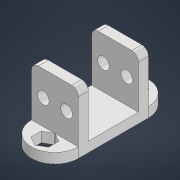
# Autodesk Inventor part: Stationary Bracket
Saved by Autodesk Inventor 2022 (Build 260153000, 153)
## iProperties
Created: 2022-01-30
Part Number: Stationary Bracket
Material: Generic
Document SubType Name: Modeling
Designer: izack
Density: 1 g/cm^3
Appearance: Default
Author: izack
## iProperties of the stored document Stationary Bracket_3DPrint.ipt
Part Number: Stationary Bracket_3DPrint
Material: Generic
Document SubType Name: Modeling
Designer: izack
Appearance: Default
Author: izack
Autodesk Inventor part; units mm, degrees
ref_plane "YZ Plane" through (0, 0, 0) normal (1, 0, 0) x (0, 1, 0)
ref_plane "XZ Plane" through (0, 0, 0) normal (0, 1, 0) x (-1, 0, 0)
ref_plane "XY Plane" through (0, 0, 0) normal (0, 0, 1) x (1, 0, 0)
sketch "Sketch1" plane through (0, 0, 0) normal (0, 1, 0) x (-1, 0, 0)
  line L0 (-7, 10.5) -> (7, 10.5)
  line L1 (7, 10.5) -> (7, -10.5)
  line L2 (7, -10.5) -> (-7, -10.5)
  line L3 (-7, -10.5) -> (-7, 10.5)
  line L4 (-7, 10.5) -> (7, -10.5) construction
  line L5 (7, 10.5) -> (-7, -10.5) construction
  line L6 (-7, 7.5) -> (7, 7.5)
  line L7 (7, 7.5) -> (7, -7.5)
  line L8 (7, -7.5) -> (-7, -7.5)
  line L9 (-7, -7.5) -> (-7, 7.5)
  line L10 (-7, 7.5) -> (7, -7.5) construction
  line L11 (7, 7.5) -> (-7, -7.5) construction
  line L12 (7, 0) -> (-7, 0) construction
  circle A0 centre (3.5, 0) radius 1.25
  circle A1 centre (-3.5, 0) radius 1.25
  point P0 (0, 0)
  dimension "d0" = 14
  dimension "d1" = 21
  dimension "d2" = 15
  dimension "d3" = 2.5
  dimension "d4" = 2.5
  dimension "d5" = 3.5
  dimension "d6" = 3.5
  constraints: 26 end point, 6 midpoint, 4 parallel, 3 point on line, 2 centre point, 2 horizontal, 2 perpendicular
  measures "d0" distance of L1.end L2.end
  measures "d1" distance of L0.end L1.end
  measures "d2" distance of L6.end L7.end
  measures "d3" diameter of A0
  measures "d4" diameter of A1
  measures "d5" distance from line of L1 A0.centre
  measures "d6" distance from line of L3 A1.centre
extrude "Extrusion1" add sketch "Sketch1" along normal blind 3
sketch "Sketch2" plane through (0, 0, 0) normal (0, -1, 0) x (1, 0, 0)
  line L0 (7, -10.5) -> (-7, -10.5) projected
  line L1 (7, 10.5) -> (7, -10.5) projected
  line L2 (-7, -10.5) -> (7, -10.5)
  line L3 (7, -10.5) -> (7, -7.5)
  line L4 (7, -7.5) -> (-7, -7.5)
  line L5 (-7, -7.5) -> (-7, -10.5)
  line L6 (-7, 10.5) -> (7, 10.5) projected
  line L7 (-7, 10.5) -> (7, 10.5)
  line L8 (7, 10.5) -> (7, 7.5)
  line L9 (7, 7.5) -> (-7, 7.5)
  line L10 (-7, 7.5) -> (-7, 10.5)
  point P0 (0, 0)
  dimension "d9" = 3
  dimension "d10" = 3
  constraints: 16 end point, 4 parallel, 2 horizontal, 2 perpendicular, 2 point on line
  measures "d9" distance of L3.end L2.end
  measures "d10" distance of L7.end L8.end
extrude "Extrusion2" add sketch "Sketch2" along normal blind 18
sketch "Sketch3" plane through (-7, 3, 10.5) normal (0, 0, 1) x (1, 0, 0)
  line L0 (14, -3) -> (0, -3) projected
  line L1 (0, -3) -> (14, -3)
  line L2 (0, -3) -> (0, -21) construction
  line L3 (0, -10.5) -> (14, -10.5) construction
  circle A0 centre (3.5, -10.5) radius 1.75
  circle A1 centre (10.5, -10.5) radius 1.75
  line L4 (14, -21) -> (14, 0) projected
  point P0 (7, -3)
  dimension "d13" = 7.5
  dimension "d14" = 3.5
  dimension "d15" = 3.5
  dimension "d16" = 3.5
  dimension "d17" = 3.5
  constraints: 4 end point, 3 point on line, 2 centre point, 1 collinear, 1 horizontal
  measures "d13" distance between parallel lines of L0 L3
  measures "d14" diameter of A0
  measures "d15" diameter of A1
  measures "d16" distance from line of L4 A1.centre
  measures "d17" distance from line of L2 A0.centre
extrude "Extrusion3" cut sketch "Sketch3" against normal through all
sketch "Sketch4" plane through (-7, 0, -7.5) normal (0, 0, 1) x (1, 0, 0)
  line L0 (0, 0) -> (0, -18) projected
  line L1 (14, 0) -> (14, -18) projected
  line L2 (0, -18) -> (14, -18)
  line L3 (14, -18) -> (14, -15)
  line L4 (14, -15) -> (0, -15)
  line L5 (0, -15) -> (0, -18)
  point P0 (7, 0)
  point P1 (0, -15)
  dimension "d20" = 3
  constraints: 8 end point, 2 parallel, 1 horizontal, 1 perpendicular, 1 point on line
  measures "d20" distance of L3.end L2.end
extrude "Extrusion4" add sketch "Sketch4" along normal up to surface (15 mm away)
sketch "Sketch5" plane through (0, -18, 0) normal (0, -1, 0) x (1, 0, 0)
  circle A0 centre (0, -13.5) radius 2.65
  circle A1 centre (0, 13.5) radius 2.65
  line L0 (7, 10.5) -> (-7, 10.5) projected
  circle A2 centre (0, 10.5) radius 7
  line L1 (-7, -10.5) -> (7, -10.5) projected
  circle A3 centre (0, -10.5) radius 7
  line L2 (-7, 10.5) -> (-7, -10.5) projected
  line L3 (-7, 10.5) -> (7, 10.5)
  line L4 (-7, -10.5) -> (7, -10.5)
  line L5 (-2.65, -11.97) -> (0, -10.44)
  line L6 (0, -10.44) -> (2.65, -11.97)
  line L7 (2.65, -11.97) -> (2.65, -15.03)
  line L8 (2.65, -15.03) -> (0, -16.56)
  line L9 (0, -16.56) -> (-2.65, -15.03)
  line L10 (-2.65, -15.03) -> (-2.65, -11.97)
  line L11 (-2.65, 15.03) -> (0, 16.56)
  line L12 (0, 16.56) -> (2.65, 15.03)
  line L13 (2.65, 15.03) -> (2.65, 11.97)
  line L14 (2.65, 11.97) -> (0, 10.44)
  line L15 (0, 10.44) -> (-2.65, 11.97)
  line L16 (-2.65, 11.97) -> (-2.65, 15.03)
  point P0 (0, 0)
  point P1 (-7, -7.5)
  point P2 (-7, 7.5)
  point P3 (-2.65, -13.5)
  point P4 (-2.65, 13.5)
  point P5 (0.1038, 10.5)
  point P6 (-0.1038, 10.5)
  point P7 (-0.1038, -10.5)
  point P8 (0.1038, -10.5)
  dimension "d23" = 5.3
  dimension "d24" = 5.3
  dimension "d25" = 6
  dimension "d26" = 6
  constraints: 28 end point, 4 midpoint, 2 coincident, 2 equal length, 2 horizontal alignment, 1 centre point, 1 point on line, 1 tangent, 33 other
  measures "d25" vertical distance of point (-7, -7.5) point (0, -13.5)
  measures "d26" vertical distance of point (0, 13.5) point (-7, 7.5)
extrude "Extrusion5" add sketch "Sketch5" against normal blind 3 contours L7 L6 L1 A3 L5 L10 L9 L8 | L13 L12 L11 L16 L15 L0 A2 L14
sketch "Sketch6" plane through (0, 3, 0) normal (0, 1, 0) x (1, 0, 0)
  line L0 (-7, 10.5) -> (-7, -10.5) projected
  line L1 (-7, -10.5) -> (7, -10.5) projected
  line L2 (-7, -10.5) -> (7, -10.5) projected
  line L3 (7, -10.5) -> (7, 10.5) projected
  line L4 (7, 10.5) -> (-7, 10.5) projected
  line L5 (-7, 10.5) -> (-7, -10.5) projected
  circle A0 centre (3.5, 0) radius 1.25 projected
  circle A1 centre (-3.5, 0) radius 1.25 projected
  point P0 (0, 0)
extrude "Extrusion6" cut sketch "Sketch6" against normal up to surface (3 mm away)
fillet "Fillet1" radius 2 4 edges at (-7, 0, -9) (7, 0, -9) (-7, 0, 9) (7, 0, 9)
body "Solid1"
